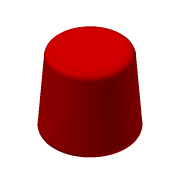
# Autodesk Inventor part: Encoder Knobe
Saved by Autodesk Inventor 2015 (Build 190159000, 159)
## iProperties
Created: 2020-02-27
Part Number: Encoder Knobe
Material: Generic
Document SubType Name: Modeling
Designer: Ghassan Yusuf
Density: 1 g/cm^3
Appearance: Default(2)
Author: Ghassan Yusuf
Autodesk Inventor part; units mm, degrees
ref_plane "YZ Plane" through (0, 0, 0) normal (1, 0, 0) x (0, 1, 0)
ref_plane "XZ Plane" through (0, 0, 0) normal (0, 1, 0) x (-1, 0, 0)
ref_plane "XY Plane" through (0, 0, 0) normal (0, 0, 1) x (1, 0, 0)
sketch "Sketch1" plane through (0, 0, 0) normal (0, 0, 1) x (1, 0, 0)
  circle A0 centre (0, 0) radius 7.5
  circle A1 centre (0, 0) radius 2.985
  dimension "d0" = 15
  dimension "d1" = 5.97
  constraints: 2 centre point, 2 coincident
  measures "d0" diameter of A0
  measures "d1" diameter of A1
extrude "Extrusion1" add sketch "Sketch1" along normal blind 14 contours A0 | A1
extrude "Extrusion2" cut sketch "Sketch1" along normal blind 10 contours A1
chamfer "Chamfer1" distance 1 distance2 13 1 edges at (-7.5, 0, 14) measured on face at (1.2064, -0.2974, 14)
fillet "Fillet1" radius 1 2 edges at (-6.5, 0, 14) (-7.5, 0, 0)
body "Solid1"
